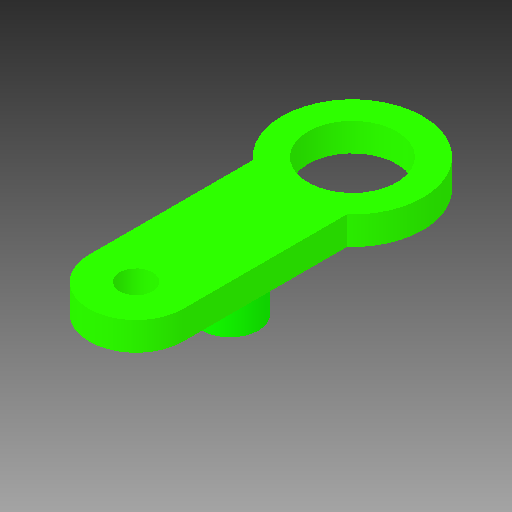
# Autodesk Inventor part: 轉軸
Saved by Autodesk Inventor 2017 (Build 210142000, 142)
## iProperties
Created: 2019-12-03
Part Number: 轉軸
Material: ABS Plastic
Document SubType Name: Modeling
Designer: 吳昇峻
Density: 1.06 g/cm^3
Appearance: Smooth - Yellow
Mass: 1.102 g
Surface Area: 10.6423 cm^2
Volume: 1.03962 cm^3
Author: 吳昇峻
Autodesk Inventor part; units mm, degrees
ref_plane "YZ Plane" through (0, 0, 0) normal (1, 0, 0) x (0, 1, 0)
ref_plane "XY Plane" through (0, 0, 0) normal (0, 0, 1) x (1, 0, 0)
sketch "草圖1" plane through (0, 0, 0) normal (0, 1, 0) x (-1, 0, 0)
  circle A0 centre (0, 0) radius 1.75
  arc A1 (5, 0) -> (-5, 0) centre (0, 0) ccw
  circle A2 centre (0, -23) radius 4.7
  arc A3 (-5, -17.4098) -> (5, -17.4098) centre (0, -23) ccw
  line L0 (-5, 0) -> (-5, -17.4098)
  line L1 (5, 0) -> (5, -17.4098)
  line L2 (0, 0) -> (0, -1.75) construction
  line L3 (0, -15.5) -> (0, -23) construction
  dimension "d0" = 3.5
  dimension "d1" = 10
  dimension "d2" = 23
  dimension "d3" = 9.4
  dimension "d4" = 15
  constraints: 8 end point, 4 coincident, 4 point on circle, 3 centre point, 3 vertical, 1 parallel, 1 vertical alignment, 2 other
  measures "d1" diameter of A1
  measures "d2" distance of L2.start L3.end
  measures "d3" diameter of A2
  measures "d4" diameter of A3
extrude "擠出1" add sketch "草圖1" along normal blind 3
ref_plane "工作平面2" through (0, 2.2, 0) normal (0, 1, 0) x (-1, 0, 0)
sketch "草圖3" plane through (0, 2.2, 0) normal (0, 1, 0) x (-1, 0, 0)
  circle A0 centre (0, -23) radius 4.7 projected
  circle A1 centre (0, 0) radius 1.75 projected
  line L0 (-5, 0) -> (-5, -17.4098) projected
  arc A2 (-5, -17.4098) -> (5, -17.4098) centre (0, -23) ccw projected
  line L1 (5, -17.4098) -> (5, 0) projected
  arc A3 (5, 0) -> (-5, 0) centre (0, 0) ccw projected
sketch "草圖4" plane through (0, 0, 0) normal (0, -1, 0) x (1, 0, 0)
  line L0 (0, 0) -> (0, -10) construction
  circle A0 centre (0, -10) radius 3
  dimension "d13" = 10
  dimension "d14" = 6
  constraints: 2 end point, 1 centre point, 1 coincident, 1 vertical
  measures "d13" distance of L0.start L0.end
  measures "d14" diameter of A0
extrude "擠出3" add sketch "草圖4" along normal blind 5
fillet "圓角1" radius 1 1 edges at (-3, 0, -10)
